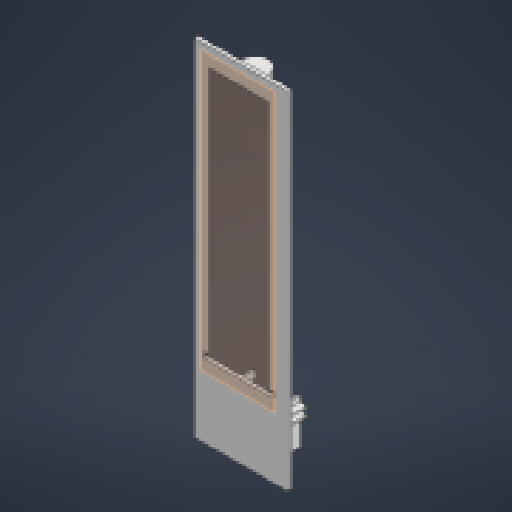
# Autodesk Inventor part: holder
Saved by Autodesk Inventor 2024.3 (Build 283343000, 343)
## iProperties
Created: 2025-08-14
Part Number: holder
Material: Generic
Document SubType Name: Modeling
Designer: giuseppe
Density: 1 g/cm^3
Appearance: Default
Author: giuseppe
Autodesk Inventor part; units mm, degrees
ref_plane "YZ Plane" through (0, 0, 0) normal (1, 0, 0) x (0, 1, 0)
ref_plane "XZ Plane" through (0, 0, 0) normal (0, 1, 0) x (-1, 0, 0)
ref_plane "XY Plane" through (0, 0, 0) normal (0, 0, 1) x (1, 0, 0)
ref_plane "Work Plane1" through (0, 0, 0) normal (0, 0, 1) x (1, 0, 0)
sketch "Sketch1" plane through (0, 0, 0) normal (0, 0, 1) x (1, 0, 0)
  line L0 (31.1769, -24.84) -> (31.1769, 108) construction
  line L1 (0, 108) -> (31.1769, 108) construction
  line L2 (0, 108) -> (0, -24.84) construction
  line L3 (-2.4511, -24.84) -> (0, -24.84) construction
  line L4 (-2.4511, -27) -> (-2.4511, -24.84) construction
  line L5 (33.628, -27) -> (-2.4511, -27) construction
  line L6 (33.628, -24.84) -> (33.628, -27) construction
  line L7 (31.1769, -24.84) -> (33.628, -24.84) construction
  line L8 (-0.5, -24.34) -> (-0.5, 108.5)
  line L9 (-0.5, 108.5) -> (31.6769, 108.5)
  line L10 (31.6769, 108.5) -> (31.6769, -24.34)
  line L11 (31.6769, -24.34) -> (34.128, -24.34)
  line L12 (34.128, -24.34) -> (34.128, -27.5)
  line L13 (34.128, -27.5) -> (-2.9511, -27.5)
  line L14 (-2.9511, -27.5) -> (-2.9511, -24.34)
  line L15 (-2.9511, -24.34) -> (-0.5, -24.34)
  line L16 (-7.9511, 118.5) -> (41.7885, 118.5)
  line L17 (41.7885, 118.5) -> (41.7885, -66.75)
  line L18 (41.7885, -66.75) -> (-7.9511, -66.75)
  line L19 (-7.9511, -66.75) -> (-7.9511, 118.5)
  line L20 (10.3385, -56.75) -> (31.1385, -56.75) construction
  line L21 (36.7885, -38.65) -> (36.7885, -41.15) construction
  line L22 (4.6885, -38.65) -> (4.6885, -41.15) construction
  point P0 (0, 0)
  dimension "d0" = 0.5
  dimension "d1" = 10
  dimension "d2" = 5
  dimension "d3" = 5
  dimension "d4" = 10
  constraints: 24 end point, 2 parallel, 1 horizontal, 1 perpendicular, 7 other
  measures "d0" distance between parallel lines of L2 L8
  measures "d1" distance between parallel lines of L18 L20
  measures "d2" distance between parallel lines of L17 L21
  measures "d3" distance between parallel lines of L14 L19
  measures "d4" distance between parallel lines of L16 L9
extrude "Extrusion1" add sketch "Sketch1" against normal blind 2
chamfer "Chamfer1" distance 1.6 angle 45 4 edges at (-0.5, 42.08, -2) (-2.9511, -25.92, -2) (31.6769, 42.08, -2) (34.128, -25.92, -2)
sketch "Sketch2" plane through (0, 0, -2) normal (0, 0, -1) x (-1, 0, 0)
  line L0 (-9.4885, -41.15) -> (-9.4885, -51.45) projected
  line L1 (-31.9885, -41.15) -> (-31.9885, -51.45) projected
  line L2 (-31.1385, -56.85) -> (-10.3385, -56.85) projected
  line L3 (-9.4885, -56.75) -> (-9.4885, -51.45) projected
  line L4 (-31.9885, -56.75) -> (-31.9885, -51.45) projected
  line L5 (-17.1505, -34.35) -> (-31.1385, -34.35) projected
  line L6 (-31.9885, -56.85) -> (-9.4885, -56.85)
  line L7 (-9.4885, -56.85) -> (-9.4885, -34.35)
  line L8 (-9.4885, -34.35) -> (-31.9885, -34.35)
  line L9 (-31.9885, -34.35) -> (-31.9885, -56.85)
  point P0 (0, 0)
  point P1 (-10.3385, -56.85)
  constraints: 8 end point, 4 collinear, 2 parallel, 1 horizontal, 1 perpendicular
ref_plane "Work Plane2" through (10.3385, -51.45, -2.9) normal (0, 0, 1) x (1, 0, 0)
extrude "Extrusion2" add sketch "Sketch2" along normal up to surface (0.9 mm away)
sketch "Sketch3" plane through (0, 0, -2) normal (0, 0, -1) x (-1, 0, 0)
  line L0 (-9.3885, -47.25) -> (-4.6885, -47.25)
  line L1 (-4.6885, -47.25) -> (-4.6885, -41.25)
  line L2 (-4.6885, -41.25) -> (-9.3885, -41.25)
  line L3 (-9.3885, -41.25) -> (-9.3885, -47.25)
  line L4 (-36.7885, -51.35) -> (-32.0885, -51.35)
  line L5 (-32.0885, -51.35) -> (-32.0885, -41.35)
  line L6 (-32.0885, -41.35) -> (-36.7885, -41.35)
  line L7 (-36.7885, -41.35) -> (-36.7885, -51.35)
  line L8 (-36.7885, -38.45) -> (-32.0885, -38.45)
  line L9 (-32.0885, -38.45) -> (-32.0885, -34.35)
  line L10 (-32.0885, -34.35) -> (-36.7885, -34.35)
  line L11 (-36.7885, -34.35) -> (-36.7885, -38.45)
  line L12 (-9.3885, -38.45) -> (-4.6885, -38.45)
  line L13 (-4.6885, -38.45) -> (-4.6885, -34.35)
  line L14 (-4.6885, -34.35) -> (-9.3885, -34.35)
  line L15 (-9.3885, -34.35) -> (-9.3885, -38.45)
  line L16 (-31.9885, -34.35) -> (-31.9885, -56.85) projected
  line L17 (-9.4885, -56.85) -> (-9.4885, -34.35) projected
  line L18 (-10.3385, -38.65) -> (-5.5385, -38.65) projected
  line L19 (-35.9385, -41.15) -> (-5.5385, -41.15) projected
  line L20 (-35.9385, -38.65) -> (-31.1385, -38.65) projected
  line L21 (-4.6885, -38.65) -> (-4.6885, -41.15) projected
  line L22 (-36.7885, -38.65) -> (-36.7885, -41.15) projected
  line L23 (-9.4885, -34.35) -> (-31.9885, -34.35) projected
  line L24 (-8.1885, -47.25) -> (-8.1885, -42.45)
  line L25 (-8.1885, -42.45) -> (-4.6885, -42.45)
  line L26 (-4.6885, -37.25) -> (-8.1885, -37.25)
  line L27 (-8.1885, -37.25) -> (-8.1885, -34.35)
  line L28 (-36.7885, -37.25) -> (-33.2885, -37.25)
  line L29 (-33.2885, -37.25) -> (-33.2885, -34.35)
  line L30 (-36.7885, -42.55) -> (-33.2885, -42.55)
  line L31 (-33.2885, -42.55) -> (-33.2885, -51.35)
  line L32 (-12.6885, -56.95) -> (-9.3885, -56.95)
  line L33 (-9.3885, -56.95) -> (-9.3885, -53.85)
  line L34 (-9.3885, -53.85) -> (-8.1885, -53.85)
  line L35 (-8.1885, -53.85) -> (-8.1885, -58.15)
  line L36 (-8.1885, -58.15) -> (-12.6885, -58.15)
  line L37 (-12.6885, -58.15) -> (-12.6885, -56.95)
  line L38 (-31.9885, -56.85) -> (-9.4885, -56.85) projected
  line L39 (-28.9885, -56.95) -> (-32.0885, -56.95)
  line L40 (-32.0885, -56.95) -> (-32.0885, -51.35)
  line L41 (-32.0885, -51.35) -> (-33.2885, -51.35)
  line L42 (-33.2885, -51.35) -> (-33.2885, -58.15)
  line L43 (-33.2885, -58.15) -> (-28.9885, -58.15)
  line L44 (-28.9885, -58.15) -> (-28.9885, -56.95)
  point P0 (0, 0)
  point P1 (-7.0385, -38.45)
  point P2 (-32.0885, -51.35)
  point P3 (-33.2885, -51.35)
  dimension "d13" = 0.1
  dimension "d14" = 0.1
  dimension "d15" = 0.1
  dimension "d16" = 0.1
  dimension "d17" = 0.1
  dimension "d18" = 0.2
  dimension "d19" = 0.2
  dimension "d20" = 0.2
  dimension "d21" = 10
  dimension "d22" = 6
  dimension "d23" = 4.7
  dimension "d24" = 1.2
  dimension "d25" = 1.2
  dimension "d26" = 1.2
  dimension "d27" = 1.2
  dimension "d28" = 1.2
  dimension "d29" = 1.2
  dimension "d30" = 1.2
  dimension "d31" = 1.2
  dimension "d32" = 1.2
  dimension "d33" = 1.2
  dimension "d34" = 0.1
  dimension "d35" = 0.1
  dimension "d36" = 4.5
  dimension "d37" = 4.3
  dimension "d38" = 1.2
  dimension "d39" = 1.2
  dimension "d40" = 0.1
  dimension "d41" = 0.1
  dimension "d42" = 4.3
  constraints: 72 end point, 22 perpendicular, 10 parallel, 9 point on line, 6 collinear, 4 horizontal, 1 midpoint
  measures "d13" distance between parallel lines of L16 L5
  measures "d14" distance between parallel lines of L16 L9
  measures "d15" distance between parallel lines of L17 L3
  measures "d16" distance between parallel lines of L17 L15
  measures "d17" distance between parallel lines of L19 L2
  measures "d18" distance between parallel lines of L18 L12
  measures "d19" distance between parallel lines of L19 L6
  measures "d20" distance between parallel lines of L20 L8
  measures "d21" distance of L6.end L4.start
  measures "d22" distance of L0.end L1.end
  measures "d23" distance of L4.start L4.end
  measures "d24" distance between parallel lines of L28 L8
  measures "d25" distance between parallel lines of L9 L29
  measures "d26" distance between parallel lines of L6 L30
  measures "d27" distance between parallel lines of L5 L31
  measures "d28" distance between parallel lines of L3 L24
  measures "d29" distance between parallel lines of L2 L25
  measures "d30" distance from line of point (-7.038, -38.45) L26
  measures "d31" distance between parallel lines of L15 L27
  measures "d32" distance of L33.end L34.end
  measures "d33" distance of L36.end L32.start
  measures "d34" distance between parallel lines of L17 L33
  measures "d35" distance between parallel lines of L38 L32
  measures "d36" distance of L35.end L36.end
  measures "d37" distance between parallel lines of L36 L34
  measures "d38" distance of L40.end L41.end
  measures "d39" distance of L43.end L39.start
  measures "d40" distance between parallel lines of L16 L40
  measures "d41" distance between parallel lines of L38 L39
  measures "d42" distance of L42.end L43.end
ref_plane "Work Plane3" through (5.5385, -41.15, -15.1) normal (0, 0, -1) x (0, 1, 0)
extrude "Extrusion3" add sketch "Sketch3" along normal up to surface (13.1 mm away) contours L3 L2 L1 L25 L24 L0 | L31 L30 L7 L6 L5 L4 | L4 L40 L39 L44 L43 L42 | L11 L28 L29 L10 L9 L8 | L15 L14 L27 L26 L13 L12 | L32 L33 L34 L35 L36 L37
sketch "Sketch5" plane through (-0.5, 108.5, 0) normal (0, -1, 0) x (1, 0, 0)
  circle A0 centre (16.0885, -9) radius 5.85 construction
  line L0 (7.0885, -2) -> (25.0885, -2)
  line L1 (-4.0511, -2) -> (36.228, -2) projected
  circle A1 centre (16.0885, -9) radius 6.85
  line L2 (7.0885, -2) -> (9.4781, -10.7959)
  line L3 (22.6989, -10.7959) -> (25.0885, -2)
  point P0 (0.5, 0)
  point P1 (16.0885, -2)
  dimension "d47" = 9
  dimension "d48" = 1
  constraints: 6 end point, 2 point on circle, 2 tangent, 1 centre point, 1 collinear, 1 horizontal, 1 midpoint, 1 vertical alignment
  measures "d47" horizontal distance of L0.start A0.centre
  measures "d48" radial gap between concentric circles of A0 A1
extrude "Extrusion4" add sketch "Sketch5" against normal blind 4
sketch "Sketch6" plane through (-0.5, 108.5, 0) normal (0, -1, 0) x (1, 0, 0)
  circle A0 centre (16.0885, -9) radius 5.85 projected
  circle A1 centre (16.0885, -9) radius 5.65
  point P0 (0.5, 0)
  dimension "d51" = 0.2
  constraints: 1 centre point
  measures "d51" radial gap between concentric circles of A0 A1
extrude "Extrusion5" add sketch "Sketch6" along normal blind 4 contours A1
body "Solid1"
